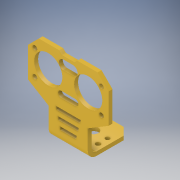
# Autodesk Inventor part: Halterung
Saved by Autodesk Inventor 2017 SP1 (Build 210196100, 196)
## iProperties
Part Number: Halterung
Material: Generisch
Document SubType Name: Blech
Designer: Alex
Density: 1 g/cm^3
Sheet Metal Rule: Standard_mm
Appearance: Vorgabe
Flat Pattern Width: 5.15 cm
Flat Pattern Length: 7.525 cm
Flat Pattern Area: 38.7538 cm^2
Sheet Metal Width: 51.500 mm
Sheet Metal Length: 75.250 mm
Sheet Metal Area: 3875.375 mm^2
Author: Alex
Autodesk Inventor part; units mm, degrees
ref_plane "YZ Plane" through (0, 0, 0) normal (1, 0, 0) x (0, 1, 0)
ref_plane "XZ Plane" through (0, 0, 0) normal (0, 1, 0) x (-1, 0, 0)
ref_plane "XY Plane" through (0, 0, 0) normal (0, 0, 1) x (1, 0, 0)
sketch "Skizze1" plane through (0, 0, 0) normal (0, 0, 1) x (1, 0, 0)
  line L0 (0, 0) -> (-4, 0)
  line L1 (-4, 0) -> (-5.75, -1.75)
  line L2 (-5.75, -1.75) -> (-18.75, -1.75)
  line L3 (-18.75, -1.75) -> (-25.75, 5.25)
  line L4 (-25.75, 5.25) -> (-25.75, 24.25)
  line L5 (-25.75, 24.25) -> (-12.5, 32.25)
  line L6 (-12.5, 32.25) -> (-12.5, 68.5)
  line L7 (-12.5, 68.5) -> (-7.5, 73.5)
  line L8 (-7.5, 73.5) -> (0, 73.5)
  line L9 (0, 0) -> (0, 73.5)
  line L10 (0, 0) -> (4, 0)
  line L11 (4, 0) -> (5.75, -1.75)
  line L12 (5.75, -1.75) -> (18.75, -1.75)
  line L13 (18.75, -1.75) -> (25.75, 5.25)
  line L14 (25.75, 5.25) -> (25.75, 24.25)
  line L15 (25.75, 24.25) -> (12.5, 32.25)
  line L16 (12.5, 32.25) -> (12.5, 68.5)
  line L17 (12.5, 68.5) -> (7.5, 73.5)
  line L18 (7.5, 73.5) -> (0, 73.5)
  dimension "d0" = 25
  dimension "d1" = 4
  dimension "d2" = 13
  dimension "d3" = 19
  dimension "d5" = 7.5
  dimension "d6" = 45
  dimension "d7" = 34
  dimension "d8" = 45
  dimension "d10" = 75.25
  dimension "d11" = 51.5
  dimension "d12" = 45
  dimension "d13" = 7
  measures "d0" diameter of L6 L9
  measures "d1" distance of L0.start L0.end
  measures "d2" distance of L1.end L2.end
  measures "d3" distance of L3.end L4.end
  measures "d5" distance of L18.start L8.end
  measures "d6" angle of L16 L17
  measures "d7" distance from line of L2 L5.end
  measures "d8" angle of L2 L3
  measures "d10" distance between parallel lines of L12 L18
  measures "d11" distance between parallel lines of L14 L4
  measures "d12" angle of L0 L1
  measures "d13" distance from line of L3.end L2
extrude "Grobblech1" add sketch "Skizze1" along normal blind 2.5
sketch "Skizze2" plane through (0, 0, 2.5) normal (0, 0, 1) x (1, 0, 0)
  line L0 (25.75, 24.25) -> (25.75, 5.25) projected
  line L1 (18.75, -1.75) -> (5.75, -1.75) projected
  line L2 (0, 48) -> (0, -16)
  point P0 (0, 0)
  point P1 (12.75, 12.25)
  point P2 (21.25, 4.75)
  point P3 (21.25, 20.75)
  point P4 (-12.75, 12.25)
  point P5 (-21.25, 4.75)
  point P6 (-21.25, 20.75)
  dimension "d15" = 16
  dimension "d16" = 8.5
  dimension "d17" = 8.5
  dimension "d18" = 4.5
  dimension "d19" = 6.5
  constraints: 3 symmetric about line, 2 end point, 1 vertical, 1 vertical alignment
  measures "d15" distance of point (21.25, 4.75) point (21.25, 20.75)
  measures "d16" horizontal distance of point (12.75, 12.25) point (21.25, 20.75)
  measures "d17" horizontal distance of point (12.75, 12.25) point (21.25, 20.75)
  measures "d18" distance from line of L0 point (21.25, 20.75)
  measures "d19" distance from line of L1 point (21.25, 4.75)
hole "Bohrung1" at (21.25, 4.75, 2.5) at (21.25, 20.75, 2.5) at (-21.25, 4.75, 2.5) at (-21.25, 20.75, 2.5) direction (0, 0, -1) diameter 3 depth 2.5 tip angle 118
hole "Bohrung2" at (12.75, 12.25, 2.5) at (-12.75, 12.25, 2.5) direction (0, 0, -1) diameter 18 depth 2.5 tip angle 118
sketch "Skizze3" plane through (0, 0, 2.5) normal (0, 0, 1) x (1, 0, 0)
  line L0 (0, -5.3655) -> (0, 31.5081)
  arc A0 (-3, 8) -> (-3, 2) centre (-3, 5) ccw
  line L1 (4, 0) -> (-4, 0) projected
  line L2 (-3, 8) -> (0, 8)
  line L3 (-3, 2) -> (0, 2)
  arc A1 (3, 2) -> (3, 8) centre (3, 5) ccw
  line L4 (3, 8) -> (0, 8)
  line L5 (3, 2) -> (0, 2)
  point P0 (0, 0)
  dimension "d34" = 3
  dimension "d35" = 6
  dimension "d36" = 5
  constraints: 10 end point, 4 point on circle, 3 symmetric about line, 2 centre point, 2 perpendicular, 2 point on line, 1 vertical, 1 other
  measures "d34" radius of A0
  measures "d35" diameter of A0.centre L0
  measures "d36" distance from line of L1 A0.centre
extrude "Ausklinkung1" cut sketch "Skizze3" against normal blind 2.5
sketch "Skizze4" plane through (0, 0, 2.5) normal (0, 0, 1) x (1, 0, 0)
  line L0 (0, 16.2064) -> (0, 31.8792)
  line L1 (4, 0) -> (-4, 0) projected
  line L2 (12.5, 68.5) -> (12.5, 32.25) projected
  arc A0 (-4.5, 24) -> (-4.5, 20) centre (-4.5, 22) ccw
  line L3 (-4.5, 24) -> (0, 24)
  line L4 (-4.5, 20) -> (0, 20)
  arc A1 (4.5, 20) -> (4.5, 24) centre (4.5, 22) ccw
  line L5 (4.5, 24) -> (0, 24)
  line L6 (4.5, 20) -> (0, 20)
  point P0 (0, 0)
  dimension "d42" = 12.5
  dimension "d43" = 2
  dimension "d44" = 9
  dimension "d45" = 22
  constraints: 10 end point, 4 point on circle, 3 symmetric about line, 2 centre point, 1 horizontal, 1 point on line, 1 vertical, 1 other
  measures "d42" distance between parallel lines of L2 L0
  measures "d43" radius of A0
  measures "d44" diameter of A0.centre L0
  measures "d45" distance from line of L1 A0.centre
extrude "Ausklinkung2" cut sketch "Skizze4" against normal blind 2.5
sketch "Skizze5" plane through (0, 0, 2.5) normal (0, 0, 1) x (1, 0, 0)
  line L0 (0, 27.2318) -> (0, 54.2603)
  line L1 (12.5, 68.5) -> (12.5, 32.25) projected
  line L2 (0, 30) -> (-8, 30)
  line L3 (-8, 30) -> (-7.5, 32)
  line L4 (-7.5, 32) -> (0, 32)
  line L5 (4, 0) -> (-4, 0) projected
  line L6 (0, 35) -> (-6.75, 35)
  line L7 (-6.75, 35) -> (-6.25, 37)
  line L8 (-6.25, 37) -> (0, 37)
  line L9 (0, 40) -> (-5.5, 40)
  line L10 (-5.5, 40) -> (-5, 42)
  line L11 (0, 30) -> (8, 30)
  line L12 (8, 30) -> (7.5, 32)
  line L13 (7.5, 32) -> (0, 32)
  line L14 (0, 35) -> (6.75, 35)
  line L15 (6.75, 35) -> (6.25, 37)
  line L16 (6.25, 37) -> (0, 37)
  line L17 (0, 40) -> (5.5, 40)
  line L18 (5.5, 40) -> (5, 42)
  line L19 (0, 42) -> (-5, 42)
  line L20 (0, 42) -> (5, 42)
  point P0 (0, 0)
  dimension "d48" = 12.5
  dimension "d49" = 30
  dimension "d50" = 2
  dimension "d52" = 3
  dimension "d54" = 3
  dimension "d55" = 2
  dimension "d57" = 7.5
  dimension "d58" = 8
  dimension "d59" = 6.75
  dimension "d60" = 6.25
  dimension "d62" = 5.5
  dimension "d65" = 75.964
  dimension "d66" = 2
  dimension "d67" = 75.964
  dimension "d68" = 75.964
  constraints: 38 end point, 6 point on line, 6 symmetric about line, 3 horizontal, 2 perpendicular, 1 vertical
  measures "d48" distance between parallel lines of L1 L0
  measures "d49" distance between parallel lines of L5 L2
  measures "d50" distance between parallel lines of L2 L4
  measures "d52" distance between parallel lines of L6 L4
  measures "d54" distance between parallel lines of L8 L9
  measures "d55" distance between parallel lines of L8 L6
  measures "d57" distance of L3.end L4.end
  measures "d58" distance of L2.start L2.end
  measures "d59" distance of L6.start L6.end
  measures "d60" distance of L7.end L8.end
  measures "d62" distance of L9.start L9.end
  measures "d65" angle of L10 L9
  measures "d66" distance between parallel lines of L9 L19
  measures "d67" angle of L7 L6
  measures "d68" angle of L3 L2
extrude "Ausklinkung3" cut sketch "Skizze5" against normal blind 2.5
sketch "Skizze6" plane through (0, 0, 2.5) normal (0, 0, 1) x (1, 0, 0)
  arc A0 (-1.35, 69.85) -> (1.35, 69.85) centre (0, 69.85) ccw
  line L0 (0, 69.85) -> (-1.35, 69.85) construction
  line L1 (0, 69.85) -> (1.35, 69.85) construction
  line L2 (0, 74) -> (0, 46)
  line L3 (12.5, 68.5) -> (12.5, 32.25) projected
  line L4 (-12.5, 32.25) -> (-12.5, 68.5) projected
  arc A1 (0, 65) -> (-3, 62) centre (0, 62) ccw
  line L5 (-7.5, 73.5) -> (7.5, 73.5) projected
  arc A2 (-7.5, 62) -> (-10.2, 62) centre (-8.85, 62) ccw
  circle A3 centre (-8.85, 55.9) radius 1.5
  line L6 (-15, 62) -> (16, 62)
  arc A4 (3, 62) -> (0, 65) centre (0, 62) ccw
  arc A5 (10.2, 62) -> (7.5, 62) centre (8.85, 62) ccw
  circle A6 centre (8.85, 55.9) radius 1.5
  arc A7 (-3, 62) -> (0, 59) centre (0, 62) ccw
  arc A8 (-10.2, 62) -> (-7.5, 62) centre (-8.85, 62) ccw
  arc A9 (7.5, 62) -> (10.2, 62) centre (8.85, 62) ccw
  arc A10 (1.35, 54.15) -> (1.35, 54.15) centre (0, 54.15) ccw
  arc A11 (0, 59) -> (3, 62) centre (0, 62) ccw
  line L7 (-1.35, 69.85) -> (-1.35, 71.85)
  line L8 (-1.35, 54.15) -> (-1.35, 52.15)
  arc A12 (1.35, 71.85) -> (-1.35, 71.85) centre (0, 71.85) ccw
  line L9 (1.35, 71.85) -> (1.35, 69.85)
  arc A13 (1.35, 54.15) -> (-1.35, 54.15) centre (0, 54.15) ccw
  arc A14 (-1.35, 52.15) -> (1.35, 52.15) centre (0, 52.15) ccw
  line L10 (1.35, 52.15) -> (1.35, 54.15)
  point P0 (0, 0)
  dimension "d72" = 1.35
  dimension "d73" = 180
  dimension "d75" = 12.5
  dimension "d78" = 3
  dimension "d81" = 11.5
  dimension "d82" = 7.85
  dimension "d83" = 90
  dimension "d84" = 1.35
  dimension "d85" = 3
  dimension "d86" = 17.6
  dimension "d99" = 8.85
  constraints: 27 point on circle, 16 end point, 15 centre point, 8 symmetric about line, 4 point on line, 2 vertical, 1 coincident, 1 horizontal alignment, 1 perpendicular, 1 vertical alignment, 7 other
  measures "d72" radius of A0
  measures "d73" angle of L0 L1
  measures "d75" distance between parallel lines of L3 L2
  measures "d78" radius of A1
  measures "d81" distance from line of A1.centre L5
  measures "d82" distance of L0.start A1.centre
  measures "d84" radius of A2
  measures "d85" diameter of A3
  measures "d86" distance from line of L5 A3.centre
  measures "d99" distance of A1.centre A2.centre
extrude "Ausklinkung4" cut sketch "Skizze6" against normal blind 2.5
sketch "Skizze7" plane through (0, 0, 2.5) normal (0, 0, 1) x (1, 0, 0)
  line L0 (-7.5, 73.5) -> (7.5, 73.5) projected
  line L1 (12.5, 68.5) -> (12.5, 32.25) projected
  line L2 (12.5, 48) -> (-12.5, 48)
  line L3 (-12.5, 32.25) -> (-12.5, 68.5) projected
  point P0 (0, 0)
  dimension "d91" = 25.5
  constraints: 2 end point, 2 point on line, 1 horizontal
  measures "d91" distance between parallel lines of L0 L2
fold "Falten1" angle 90 bend radius 3 thickness 2.5 k factor 0.44 line from (12.5, 48, 2.5) to (-12.5, 48, 2.5) line at bend centre moving side (0, -1, 0) folds toward (0, 0, 1)
equation "\"d25\" = Stärke"
equation "\"d32\" = Stärke"
equation "\"d37\" = Stärke"
equation "\"d46\" = Stärke"
equation "\"Biegeradius\" = Stärke"
equation "\"BreiteBiegungsfreistellung\" = Stärke"
equation "\"TiefeBiegungsfreistellung\" = 0.5 * Stärke"
equation "\"MinimalRest\" = 2 * Stärke"
equation "\"Übergangsradius\" = Biegeradius"
equation "\"JacobiRadiusGröße\" = Biegeradius"
equation "\"Abstandsgröße\" = Stärke"
equation "\"d14\" = Biegeradius"
equation "\"Stärke\" = 2.5"
